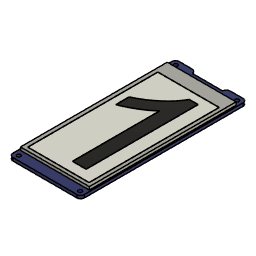
29_epaper_4_digit v15 (Autodesk Fusion 360 archive; units mm, degrees)
design "29epaper"
Autodesk Fusion 360 part; units mm, degrees
sketch "Skizze1" plane through (0, 0, 0) normal (0, 0, 1) x (1, 0, 0)
  line L0 (-16.5, 42.25) -> (16.5, 42.25) construction
  line L1 (16.5, 42.25) -> (16.5, -42.25) construction
  line L2 (16.5, -42.25) -> (-16.5, -42.25) construction
  line L3 (-16.5, -42.25) -> (-16.5, 42.25) construction
  line L4 (0, 0) -> (16.5, 0) construction
  line L5 (0, 0) -> (0, 42.25) construction
  line L6 (-19.25, 44.75) -> (19.25, 44.75)
  line L7 (19.25, 44.75) -> (19.25, -44.75)
  line L8 (19.25, -44.75) -> (-19.25, -44.75)
  line L9 (-19.25, -44.75) -> (-19.25, 44.75)
  line L10 (-16.5, 32.55) -> (16.5, 32.55)
  line L11 (16.5, 32.55) -> (16.5, -37.45)
  line L12 (16.5, -37.45) -> (-16.5, -37.45)
  line L13 (-16.5, -37.45) -> (-16.5, 32.55)
  line L14 (-18.5, 39.65) -> (18.5, 39.65)
  line L15 (18.5, 39.65) -> (18.5, -39.35)
  line L16 (18.5, -39.35) -> (-18.5, -39.35)
  line L17 (-18.5, -39.35) -> (-18.5, 39.65)
  line L18 (-8.9375, 44.75) -> (-8, 42.75)
  line L19 (-8, 42.75) -> (8, 42.75)
  line L20 (8, 42.75) -> (8.9375, 44.75)
  dimension "d1" = 33
  dimension "d2" = 84.5
  dimension "d3" = 38.5
  dimension "d4" = 89.5
  dimension "d5" = 33
  dimension "d6" = 70
  dimension "d7" = 12.2
  dimension "d8" = 37
  dimension "d9" = 79
  dimension "d10" = 5.4
  dimension "d20" = 17.875
  dimension "d21" = 2
  dimension "d22" = 16
  constraint horizontal L0
  constraint vertical L1
  constraint horizontal L2
  constraint vertical L3
  constraint coincident L4.start L5.start
  constraint midpoint L1 L4.end
  constraint midpoint L0 L5.end
  constraint vertical L5
  constraint horizontal L4
  constraint horizontal L6
  constraint vertical L7
  constraint horizontal L8
  constraint vertical L9
  constraint symmetric L4 L6 L8
  constraint symmetric L5 L7 L9
  constraint horizontal L10
  constraint vertical L11
  constraint horizontal L12
  constraint vertical L13
  constraint symmetric L5 L11 L13
  constraint horizontal L14
  constraint vertical L15
  constraint horizontal L16
  constraint vertical L17
  constraint symmetric L5 L15 L17
  constraint parallel L0 L19
  constraint coincident L6 L20.end
  constraint symmetric L5 L18.end L19.end
  constraint symmetric L5 L18 L20
  constraint coincident L6 L18.start
  measures "d1" distance of L0.start L0.end
  measures "d2" distance of L0.end L1.end
  measures "d3" distance of L6.start L6.end
  measures "d4" distance of L6 L8
  measures "d5" distance of L10.start L10.end
  measures "d6" distance of L10 L12
  measures "d7" distance of L6 L10
  measures "d8" distance of L15 L17
  measures "d9" distance of L14 L16
  measures "d10" distance of L8 L16
  measures "d20" horizontal distance of L18.start L20.end
  measures "d21" distance of L6 L19
  measures "d22" distance of L18.end L19.end
extrude "Extrusion1" add sketch "Skizze1" against normal blind 1.6 contours L6 L7 L8 L9 L18 L19 L20 | L10 L11 L12 L13 | L14 L15 L16 L17 makes body 1
extrude "Extrusion2" add sketch "Skizze1" along normal blind 1.6 separate body contours L10 L11 L12 L13 | L14 L15 L16 L17 makes body 2
extrude "Extrusion3" cut sketch "Skizze1" against normal blind 0.1 from surface at 1.6 contours L10 L11 L12 L13 bodies 2
fillet "Abrundung1" radius 2 6 edges at (19.25, -44.75, -0.8) (-19.25, -44.75, -0.8) (-19.25, 44.75, -0.8) (19.25, 44.75, -0.8) (-8.9375, 44.75, -0.8) (8.9375, 44.75, -0.8) on bodies 1
hole "Bohrung1" at (-16.5, -42.25, 0) at (16.5, -42.25, 0) at (16.5, 42.25, 0) at (-16.5, 42.25, 0) direction (0, 0, -1) diameter 2 end through all bodies 1
sketch "Skizze2" plane through (0, 0, 1.5) normal (0, 0, 1) x (-1, 0, 0)
  line L0 (16.5, -32.55) -> (16.5, 37.45)
  line L1 (16.5, 37.45) -> (-16.5, 37.45)
  line L2 (-16.5, 37.45) -> (-16.5, -32.55)
  line L3 (-16.5, -32.55) -> (16.5, -32.55)
  line L4 (12.6187, 32.0053) -> (-13.3813, 32.0053) construction
  line L5 (-13.3813, 32.0053) -> (-13.3813, -27.9947) construction
  line L6 (-13.3813, -27.9947) -> (12.6187, -27.9947) construction
  line L7 (12.6187, -27.9947) -> (12.6187, 32.0053) construction
  dimension "d25" = 60
  text T0 "1" font "Arial" height 60 align left top in box 26 x 60 at (12.6187, 32.0053) x (-1, 0) y (0, -1) spacing 1 kerned
extrude "Extrusion4" add sketch "Skizze2" along normal blind 0.1 text T0 bodies 2
equation "d2 = 86.5 mm - 2 mm"
equation "d13 = 3.2 mm - 1.6 mm"

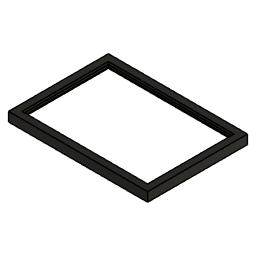
design "ikea_roederalm"
Autodesk Fusion 360 part; units mm, degrees
sketch "Skizze1" plane through (0, 0, 0) normal (0, 0, 1) x (1, 0, 0)
  line L0 (-151.5, 106.5) -> (151.5, 106.5)
  line L1 (151.5, 106.5) -> (151.5, -106.5)
  line L2 (151.5, -106.5) -> (-151.5, -106.5)
  line L3 (-151.5, -106.5) -> (-151.5, 106.5)
  line L4 (-159.3, 114.3) -> (159.3, 114.3)
  line L5 (159.3, 114.3) -> (159.3, -114.3)
  line L6 (159.3, -114.3) -> (-159.3, -114.3)
  line L7 (-159.3, -114.3) -> (-159.3, 114.3)
  line L8 (-148.5, 104) -> (148.5, 104)
  line L9 (148.5, 104) -> (148.5, -104)
  line L10 (148.5, -104) -> (-148.5, -104)
  line L11 (-148.5, -104) -> (-148.5, 104)
  line L12 (-144, 99) -> (144, 99)
  line L13 (144, 99) -> (144, -99)
  line L14 (144, -99) -> (-144, -99)
  line L15 (-144, -99) -> (-144, 99)
  line L16 (0, 0) -> (0, 106.5) construction
  line L17 (0, 0) -> (151.5, 0) construction
  dimension "d1" = 7.8
  dimension "d2" = 7.8
  dimension "d3" = 7.8
  dimension "d4" = 7.8
  dimension "d5" = 303
  dimension "d6" = 213
  dimension "d7" = 297
  dimension "d8" = 208
  dimension "d9" = 288
  dimension "d10" = 198
  constraint horizontal L0
  constraint vertical L1
  constraint horizontal L2
  constraint vertical L3
  constraint horizontal L4
  constraint vertical L5
  constraint horizontal L6
  constraint vertical L7
  constraint horizontal L8
  constraint vertical L9
  constraint horizontal L10
  constraint vertical L11
  constraint horizontal L12
  constraint vertical L13
  constraint horizontal L14
  constraint vertical L15
  constraint coincident L16.start L17.start
  constraint perpendicular L4 L16
  constraint perpendicular L16 L17
  constraint coincident L0 L16.end
  constraint symmetric L1 L3 L16
  constraint symmetric L0 L2 L17
  constraint coincident L1 L17.end
  constraint symmetric L12 L14 L17
  constraint symmetric L9 L11 L16
  constraint symmetric L13 L15 L16
  constraint symmetric L8 L10 L17
  measures "d1" distance of L3 L7
  measures "d2" distance of L0 L4
  measures "d3" distance of L1 L5
  measures "d4" distance of L2 L6
  measures "d5" distance of L1 L3
  measures "d6" distance of L0 L2
  measures "d7" distance of L8.start L8.end
  measures "d8" distance of L8.end L9.end
  measures "d9" distance of L12.start L12.end
  measures "d10" distance of L12.start L14.end
extrude "Extrusion1" add sketch "Skizze1" along normal blind 6 contours L0 L1 L2 L3 | L4 L5 L6 L7 | L8 L9 L10 L11 makes body 1
extrude "Extrusion2" add sketch "Skizze1" against normal blind 6 from surface at -4 separate body contours L0 L1 L2 L3 makes body 2
extrude "Extrusion3" add sketch "Skizze1" against normal blind 15 contours L4 L5 L6 L7 bodies 1 2
equation "d2 = d1"
equation "d3 = d1"
equation "d4 = d1"
